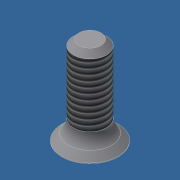
# Autodesk Inventor part: ISO14581_M3x8
Saved by Autodesk Inventor 2019 (Build 230136000, 136)
## iProperties
Created: 2019-09-01
Part Number: ISO14581_M3x8
Material: Acier zingué, clair
Description: Vis t co à 6 lobes internes
Document SubType Name: Modeling
Designer: JVY
Authority: BN4851
Density: 7.85 g/cm^3
Appearance: Par défaut
Mass: 0.291708 g
Surface Area: 0.91399 cm^2
Volume: 0.0371603 cm^3
Material number: ---
Author: JVY
Autodesk Inventor part; units mm, degrees
ref_plane "Plan YZ" through (0, 0, 0) normal (1, 0, 0) x (0, 1, 0)
ref_plane "Plan XZ" through (0, 0, 0) normal (0, 1, 0) x (-1, 0, 0)
ref_plane "Plan XY" through (0, 0, 0) normal (0, 0, 1) x (1, 0, 0)
sketch "Esquisse6" plane through (0, 0, 0) normal (0, 1, 0) x (-1, 0, 0)
  line L0 (0, 0) -> (2.548, 0)
  line L1 (2.548, 0.05) -> (1.9686, 0.6294)
  line L2 (1.5, 1.7607) -> (1.5, 7.5)
  line L3 (1, 8) -> (0, 8)
  line L4 (0, -1.6) -> (0, 9.6) construction
  line L5 (2.548, 0) -> (2.548, 0.05)
  arc A0 (1.5, 1.7607) -> (1.9686, 0.6294) centre (3.1, 1.7607) ccw
  line L6 (1.5, 7.5) -> (1, 8)
  line L7 (0, 0.6997) -> (1.4, 0.6997)
  line L8 (1.4, 0.6997) -> (0, 1.508)
  line L9 (0, 8) -> (0, 1.508)
  line L10 (0, 0.6997) -> (0, 0)
  point P0 (1.5, 8)
  dimension "d9" = 5.096
  dimension "d10" = 45
  dimension "d11" = 0.05
  dimension "d12" = 1.6
  dimension "d13" = 8
  dimension "d14" = 3
  dimension "d16" = 0.5
  dimension "d17" = 0.5
  dimension "d36" = 60
  dimension "d37" = 1.508
  dimension "d38" = 2.8
  constraints: 20 end point, 5 point on line, 3 horizontal, 2 parallel, 2 point on circle, 2 tangent, 1 centre point, 1 perpendicular, 1 vertical
  measures "d9" diameter of L0.end L4
  measures "d10" angle of L5 L1
  measures "d11" distance of L0.end L1.start
  measures "d12" radius of A0
  measures "d13" distance from line of L3 point (0, 0)
  measures "d14" diameter of L2 L4
  measures "d16" distance of L2.end point (1.5, 8)
  measures "d17" distance of L3.start point (1.5, 8)
  measures "d36" angle of L4 L8
  measures "d37" distance from line of L0 L8.end
  measures "d38" diameter of L7.end L4
revolve "Révolution1" add sketch "Esquisse6" angle 360 about axis through (0, 0, 0) along (0, 0, 1)
sketch "Esquisse1" plane through (0, 0, 0) normal (0, 0, 1) x (1, 0, 0)
  circle A0 centre (0, 0) radius 1.15 construction
  line L0 (1.299, 2.25) -> (0, 0) construction
  line L1 (0, 3.0788) -> (0, -2.723) construction
  circle A1 centre (0, 1.15) radius 0.25 construction
  circle A2 centre (0.7761, 1.3442) radius 0.55 construction
  circle A3 centre (-0.9959, 0.575) radius 0.25 construction
  circle A4 centre (-0.7761, 1.3442) radius 0.55 construction
  circle A5 centre (-0.9959, -0.575) radius 0.25 construction
  circle A6 centre (-1.5521, 0) radius 0.55 construction
  circle A7 centre (0, -1.15) radius 0.25 construction
  circle A8 centre (-0.7761, -1.3442) radius 0.55 construction
  circle A9 centre (0.9959, -0.575) radius 0.25 construction
  circle A10 centre (0.7761, -1.3442) radius 0.55 construction
  circle A11 centre (0.9959, 0.575) radius 0.25 construction
  circle A12 centre (1.5521, 0) radius 0.55 construction
  arc A13 (0.2425, 1.2107) -> (-0.2425, 1.2107) centre (0, 1.15) ccw
  arc A14 (-0.9272, 0.8154) -> (-0.2425, 1.2107) centre (-0.7761, 1.3442) ccw
  arc A15 (-0.9272, 0.8154) -> (-1.1697, 0.3953) centre (-0.9959, 0.575) ccw
  arc A16 (-1.1697, -0.3953) -> (-1.1697, 0.3953) centre (-1.5521, 0) ccw
  arc A17 (-1.1697, -0.3953) -> (-0.9272, -0.8154) centre (-0.9959, -0.575) ccw
  arc A18 (-0.2425, -1.2107) -> (-0.9272, -0.8154) centre (-0.7761, -1.3442) ccw
  arc A19 (-0.2425, -1.2107) -> (0.2425, -1.2107) centre (0, -1.15) ccw
  arc A20 (0.9272, -0.8154) -> (0.2425, -1.2107) centre (0.7761, -1.3442) ccw
  arc A21 (0.9272, -0.8154) -> (1.1697, -0.3953) centre (0.9959, -0.575) ccw
  arc A22 (1.1697, 0.3953) -> (1.1697, -0.3953) centre (1.5521, 0) ccw
  arc A23 (1.1697, 0.3953) -> (0.9272, 0.8154) centre (0.9959, 0.575) ccw
  arc A24 (0.2425, 1.2107) -> (0.9272, 0.8154) centre (0.7761, 1.3442) ccw
  circle A25 centre (0, 0) radius 1.4 construction
  dimension "d4" = 2.3
  dimension "d2" = 30
  dimension "d18" = 0.5
  dimension "d19" = 1.1
  dimension "d25" = 360
  dimension "d39" = 2.8
  constraints: 25 centre point, 24 point on circle, 14 concentric, 14 tangent, 2 coincident, 2 end point, 2 point on line, 1 vertical alignment, 27 other
  measures "d2" angle of L1 L0
  measures "d18" diameter of A1
  measures "d19" diameter of A2
  measures "d39" diameter of A25
extrude "Extrusion2" cut sketch "Esquisse1" along normal up to next
thread "Filetage1" size "M3x0.5" class "6g" standard "ANSI Metric M Profile" full length
equation "\"d17\" = d16"
equation "\"d38\" = d39"
